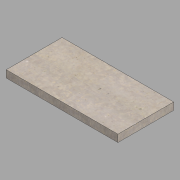
# Autodesk Inventor part: Paver type 1-pedestrian
Saved by Autodesk Inventor 2022 (Build 260153000, 153)
## iProperties
Created: 2021-10-21
Part Number: Paver type 1-pedestrian
Material: Limestone
Document SubType Name: Modeling
Designer: awelt
Density: 2.6 g/cm^3
Appearance: Kasota Gray
Author: awelt
Autodesk Inventor part; units mm, degrees
ref_plane "YZ Plane" through (0, 0, 0) normal (1, 0, 0) x (0, 1, 0)
ref_plane "XZ Plane" through (0, 0, 0) normal (0, 1, 0) x (-1, 0, 0)
ref_plane "XY Plane" through (0, 0, 0) normal (0, 0, 1) x (1, 0, 0)
sketch "Sketch1" plane through (0, 0, 0) normal (0, 1, 0) x (-1, 0, 0)
  line L0 (609.6, -304.8) -> (-609.6, -304.8)
  line L1 (-609.6, -304.8) -> (-609.6, 304.8)
  line L2 (-609.6, 304.8) -> (609.6, 304.8)
  line L3 (609.6, 304.8) -> (609.6, -304.8)
  line L4 (609.6, -304.8) -> (-609.6, 304.8) construction
  line L5 (-609.6, -304.8) -> (609.6, 304.8) construction
  point P0 (0, 0)
  dimension "d0" = 1219.2
  dimension "d1" = 609.6
  constraints: 12 end point, 2 midpoint, 2 parallel, 1 horizontal, 1 perpendicular
  measures "d0" distance of L1.end L2.end
  measures "d1" distance of L0.end L1.end
extrude "Extrusion1" add sketch "Sketch1" along normal blind 79.375
